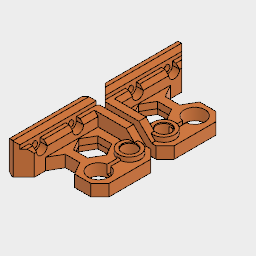
z_top_fix_v2.1 (Autodesk Fusion 360 design; units mm, degrees)
Autodesk Fusion 360 part; units mm, degrees
note: some values were not read from the file. Chosen so that the rebuilt part matches the saved one: which sketch regions a step uses; a direction; which face or edge a step refers to.
sketch "base_top_holes" plane through (0, 0, 0) normal (0, 0, 1) x (1, 0, 0)
  line L0 (0, 0) -> (38, 0)
  line L1 (38, 0) -> (38, 33)
  line L2 (8, 45) -> (0, 45)
  line L3 (0, 45) -> (0, 0)
  line L4 (8, 45) -> (8, 0)
  line L5 (8, 4) -> (30.5, 4)
  circle A0 centre (29.3, 8) radius 4
  circle A1 centre (16, 15) radius 7.7 construction
  circle A2 centre (16, 33) radius 8 construction
  circle A3 centre (29.3, 25) radius 5.75
  line L6 (16, 15) -> (16, 33) construction
  line L7 (29.3, 8) -> (29.3, 25) construction
  line L8 (20, 39.9282) -> (12, 39.9282)
  line L9 (12, 39.9282) -> (8, 33)
  line L10 (8, 33) -> (12, 26.0718)
  line L11 (12, 26.0718) -> (20, 26.0718)
  line L12 (20, 26.0718) -> (24, 33)
  line L13 (24, 33) -> (20, 39.9282)
  line L14 (23.7, 15) -> (19.85, 21.6684)
  line L15 (19.85, 21.6684) -> (12.15, 21.6684)
  line L16 (12.15, 21.6684) -> (8.3, 15)
  line L17 (8.3, 15) -> (12.15, 8.3316)
  line L18 (12.15, 8.3316) -> (19.85, 8.3316)
  line L19 (19.85, 8.3316) -> (23.7, 15)
  line L20 (28.3, 23) -> (30.3, 23)
  line L21 (30.3, 23) -> (30.3, 8)
  line L22 (30.3, 8) -> (28.3, 8)
  line L23 (28.3, 8) -> (28.3, 23)
  line L24 (30.5, 4) -> (30.5, 0)
  circle A4 centre (29.3, 8) radius 2.5
  line L25 (38, 33) -> (8, 33)
  line L26 (4, 0) -> (4, 45)
  point P0 (16, 33)
  point P1 (16, 15)
  dimension "d1" = 38
  dimension "d2" = 45
  dimension "d3" = 8
  dimension "d5" = 8
  dimension "d6" = 29.3
  dimension "d7" = 8
  dimension "d8" = 16
  dimension "d9" = 15
  dimension "d10" = 33
  dimension "d11" = 25
  dimension "d12" = 16
  dimension "d13" = 15.4
  dimension "d14" = 11.5
  dimension "d15" = 15
  dimension "d16" = 2
  dimension "d17" = 4
  dimension "d18" = 7.5
  dimension "d41" = 1.5
  measures "d1" distance of L0.start L0.end
  measures "d2" distance of L0.start L2.end
  measures "d3" distance of L2.end L2.start
  measures "d5" diameter of A0
  measures "d6" distance of L3 A0.centre
  measures "d7" distance of L0.start A0.centre
  measures "d8" distance of L0.start P1
  measures "d9" distance of L0.start P1
  measures "d10" distance of L0.start A2.centre
  measures "d11" distance of L0.start A3.centre
  measures "d12" diameter of A2
  measures "d13" diameter of A1
  measures "d14" diameter of A3
  measures "d15" distance of L20.end L21.end
  measures "d16" distance of L21.end L22.end
  measures "d17" distance of L5.end L24.end
  measures "d18" distance of L1 L24
  measures "d41" distance of A0 A4
extrude "Extrude1" add sketch "base_top_holes" against normal blind 6.5 contours L0 L2 L3 L26 | L0 L2 L4 L26 | L0 L4 L5 L24 | L0 L1 L4 L5 L10 L11 L12 L24 L25 makes body 1
extrude "Extrude2" add sketch "base_top_holes" along normal blind 11 contours L0 L2 L3 L26 bodies 1
extrude "Extrude3" add sketch "base_top_holes" along normal blind 7 contours L0 L2 L4 L26 | L0 L4 L5 L24 bodies 1
extrude "Extrude7" add sketch "base_top_holes" along normal blind 1.5 from surface at -6.5 contours A0 L21 L23 A4 | A0 A3 L21 L23 | A0 L21 L23 A4 bodies 1
sketch "frame_holes" plane through (0, 0, 0) normal (-1, 0, 0) x (0, -1, 0)
  line L0 (-45, 11) -> (-45, -6.5)
  line L1 (-45, -6.5) -> (0, -6.5)
  line L2 (0, -6.5) -> (0, 11)
  line L3 (0, 11) -> (-45, 11)
  line L4 (0, -6.5) -> (-45, -6.5)
  line L5 (0, -6.5) -> (0, 11)
  circle A0 centre (-15, 5) radius 3
  circle A1 centre (-35, 5) radius 3
  circle A2 centre (-35, 5) radius 1.65
  circle A3 centre (-15, 5) radius 1.65
  line L6 (-35, 5) -> (-15, 5) construction
  line L7 (0, 7) -> (-45, 7)
  line L8 (0, 7) -> (-45, 7)
  line L9 (-45, 7) -> (-45, 11)
  line L10 (-45, 11) -> (0, 11)
  line L11 (0, 11) -> (0, 7)
  line L12 (-38, 7) -> (-38, 5)
  line L13 (-32, 5) -> (-32, 7)
  line L14 (-18, 5) -> (-18, 7)
  line L15 (-12, 5) -> (-12, 7)
  line L16 (-35.825, 6.4289) -> (-35.4039, 6.85)
  line L17 (-35.4039, 6.85) -> (-34.5961, 6.85)
  line L18 (-34.5961, 6.85) -> (-34.175, 6.4289)
  line L19 (-15.825, 6.4289) -> (-15.4039, 6.85)
  line L20 (-15.4039, 6.85) -> (-14.5961, 6.85)
  line L21 (-14.5961, 6.85) -> (-14.175, 6.4289)
  line L22 (-35, 6.85) -> (-35, 5) construction
  line L23 (-15, 6.85) -> (-15, 5) construction
  dimension "d26" = 3.3
  dimension "d27" = 3.3
  dimension "d28" = 15
  dimension "d29" = 20
  dimension "d30" = 11.5
  dimension "d31" = 6
  dimension "d32" = 6
  dimension "d123" = 0.2
  dimension "d124" = 45
  dimension "d125" = 1.65
  dimension "d126" = 0.2
  dimension "d128" = 1.65
  measures "d26" diameter of A2
  measures "d27" diameter of A3
  measures "d28" distance of L1.end A0.centre
  measures "d29" distance of A0.centre A1.centre
  measures "d30" distance of L1.end A0.centre
  measures "d31" diameter of A1
  measures "d32" diameter of A0
  measures "d123" distance of A2 L17
  measures "d124" angle of L16 L17
  measures "d125" distance of L16.start L18.end
  measures "d126" distance of A3 L20
  measures "d128" distance of L19.start L21.end
extrude "Extrude5" cut sketch "frame_holes" against normal up to surface (8 mm away) contours A1 L7 L8 L12 | A1 L7 L8 | A1 L7 L8 | A0 L7 L8 L15 | A1 L7 L8 L13 | A0 L7 L8 | A0 L7 L8 | A0 L7 L8 L14 | A2 | A2 L16 L17 L18 | A3 | A3 L19 L20 L21 bodies 1
extrude "Extrude6" add sketch "frame_holes" against normal blind 4 contours A1 L7 L8 L12 | A1 L7 L8 | A1 L7 L8 | A0 L7 L8 L15 | A1 L7 L8 L13 | A0 L7 L8 | A0 L7 L8 | A0 L7 L8 L14 bodies 1
chamfer "Chamfer1" distance 2 angle 45 4 edges at (8, 8, 7) (8, 25, 7) (8, 41.5, 7) (4, 22.5, 11) on bodies 1
chamfer "Chamfer2" distance 7 angle 45 1 edges at (30.5, 2, 7) on bodies 1
chamfer "Chamfer3" distance 5 angle 45 2 edges at (38, 33, -3.25) (38, 0, -3.25) on bodies 1
chamfer "Chamfer4" distance 5.8 angle 45 1 edges at (8, 45, -0.75) on bodies 1
sketch "chamfer_line" plane through (0, 0, 0) normal (-1, 0, 0) x (0, -1, 0)
  line L0 (-45, 11) -> (-45, -6.5)
  line L1 (-45, -6.5) -> (0, -6.5)
  line L2 (0, -6.5) -> (0, 11)
  line L3 (0, 11) -> (-45, 11)
  line L4 (0, -6.5) -> (0, 11)
  line L5 (0, -6.5) -> (-45, -6.5)
  line L6 (-11.5, -6.5) -> (0, 5)
  arc A0 (-35.825, 6.4289) -> (-34.175, 6.4289) centre (-35, 5) ccw
  line L7 (-35.825, 6.4289) -> (-35.4039, 6.85)
  line L8 (-35.4039, 6.85) -> (-34.5961, 6.85)
  line L9 (-34.5961, 6.85) -> (-34.175, 6.4289)
  arc A1 (-15.825, 6.4289) -> (-14.175, 6.4289) centre (-15, 5) ccw
  line L10 (-15.825, 6.4289) -> (-15.4039, 6.85)
  line L11 (-15.4039, 6.85) -> (-14.5961, 6.85)
  line L12 (-14.5961, 6.85) -> (-14.175, 6.4289)
  dimension "d58" = 11.5
  dimension "d59" = 11.5
  measures "d58" distance of L1.end L6.start
  measures "d59" distance of L1.end L6.end
ref_plane "WorkPlane1" through (0, 5.75, -0.75) normal (-0.707107, 0.5, 0.5) x (0, -0.707107, 0.707107)
sketch "chamfer" plane through (0, 5.75, -0.75) normal (-0.707107, 0.5, 0.5) x (0, -0.707107, 0.707107)
  line L0 (0, -5.75) -> (12.3744, 3)
  line L1 (0, -5.75) -> (-31.8198, 16.75)
  line L2 (-8.1317, 0) -> (8.1317, 0)
  point P0 (8.1317, 0)
extrude "Extrude8" cut sketch "chamfer" against normal blind 30 bodies 1
sketch "rod_reinforcement" plane through (0, 0, 0) normal (0, 0, 1) x (-1, 0, 0)
  line L0 (-33, 0) -> (-38, -5)
  line L1 (-38, -5) -> (-38, -28)
  line L2 (-38, -28) -> (-33, -33)
  line L3 (-33, -33) -> (-24, -33)
  line L4 (-24, -33) -> (-20, -26.0718)
  line L5 (-20, -26.0718) -> (-12, -26.0718)
  line L6 (-12, -26.0718) -> (-8, -33)
  line L7 (-8, -33) -> (-8, -4)
  line L8 (-8.3, -15) -> (-12.15, -21.6684)
  line L9 (-12.15, -21.6684) -> (-19.85, -21.6684)
  line L10 (-19.85, -21.6684) -> (-23.7, -15)
  line L11 (-23.7, -15) -> (-19.85, -8.3316)
  line L12 (-19.85, -8.3316) -> (-12.15, -8.3316)
  line L13 (-12.15, -8.3316) -> (-8.3, -15)
  line L14 (-8, -4) -> (-29.3, -4)
  arc A0 (-28.3, -11.873) -> (-29.3, -4) centre (-29.3, -8) ccw
  line L15 (-28.3, -11.873) -> (-28.3, -19.3376)
  arc A1 (-30.3, -19.3376) -> (-28.3, -19.3376) centre (-29.3, -25) ccw
  line L16 (-30.3, -19.3376) -> (-30.3, -11.873)
  arc A2 (-29.3, -4) -> (-30.3, -11.873) centre (-29.3, -8) ccw
  line L17 (-30.5, -4) -> (-30.5, 0)
  line L18 (-30.5, 0) -> (-33, 0)
  arc A3 (-30.3, -19.3376) -> (-28.3, -19.3376) centre (-29.3, -25) ccw
  line L19 (-38, -5) -> (-38, -28)
  circle A4 centre (-29.3, -8) radius 6
  line L20 (-30.3, -19.3376) -> (-30.3, -11.873)
  line L21 (-28.3, -11.873) -> (-28.3, -19.3376)
  arc A5 (-28.3, -11.873) -> (-29.3, -4) centre (-29.3, -8) ccw
  arc A6 (-29.3, -4) -> (-30.3, -11.873) centre (-29.3, -8) ccw
  circle A7 centre (-29.3, -8) radius 2.5
  arc A8 (-30.3, -11.873) -> (-28.3, -11.873) centre (-29.3, -8) ccw
  line L22 (-29.3, -4) -> (-30.5, -4)
  dimension "d76" = 12
  measures "d76" diameter of A4
extrude "Extrude11" add sketch "rod_reinforcement" along normal blind 2.5 contours L14 L17 A4 L22 | L16 A2 L17 A4 L20 A6 L22 | L14 A0 L15 A4 L21 A5 bodies 1
extrude "Extrude12" add sketch "rod_reinforcement" against normal blind 1.6 from surface at 2.5 contours L14 L17 A4 L22 | L15 L16 A4 L20 L21 A8 bodies 1
chamfer "Chamfer11" distance 0.5 distance2 0.15 1 edges at (29.7682, 4.0275, 2.5) measured on face at (30.6677, 11.7589, 1.1333) on bodies 1
chamfer "Chamfer6" distance 5 angle 45 1 edges at (0, 0, 8) on bodies 1
chamfer "Chamfer9" distance 1.5 angle 45 1 edges at (0, 28.25, -6.5) on bodies 1
chamfer "Chamfer10" distance 0.26 distance2 3 6 edges at (10.225, 18.3342, -6.5) (10.225, 11.6658, -6.5) (16, 8.3316, -6.5) (21.775, 11.6658, -6.5) (21.775, 18.3342, -6.5) (16, 21.6684, -6.5) measured on face at (3.6667, 29.1262, -6.5) measured on face at (3.6667, 29.1262, -6.5) measured on face at (3.6667, 29.1262, -6.5) measured on face at (3.6667, 29.1262, -6.5) measured on face at (3.6667, 29.1262, -6.5) measured on face at (3.6667, 29.1262, -6.5) on bodies 1
sketch "selective_infill" plane through (0, 0, -6.5) normal (0, 0, -1) x (1, 0, 0)
  circle A0 centre (29.3, -8) radius 2.5
  circle A1 centre (29.3, -25) radius 5.75
  line L0 (1.5, -9.3787) -> (1.5, -45)
  line L1 (1.5, -45) -> (2.2, -45)
  line L2 (2.2, -45) -> (8, -39.2)
  line L3 (8, -39.2) -> (8, -33)
  line L4 (8, -33) -> (12, -26.0718)
  line L5 (12, -26.0718) -> (20, -26.0718)
  line L6 (20, -26.0718) -> (24, -33)
  line L7 (24, -33) -> (33, -33)
  line L8 (33, -33) -> (38, -28)
  line L9 (38, -28) -> (38, -5)
  line L10 (38, -5) -> (33, 0)
  line L11 (33, 0) -> (8.1317, 0)
  line L12 (8.1317, 0) -> (1.5, -9.3787)
  line L13 (20.0001, -8.0716) -> (24.0002, -15)
  line L14 (24.0002, -15) -> (20.0001, -21.9284)
  line L15 (20.0001, -21.9284) -> (11.9999, -21.9284)
  line L16 (11.9999, -21.9284) -> (7.9998, -15)
  line L17 (7.9998, -15) -> (11.9999, -8.0716)
  line L18 (11.9999, -8.0716) -> (20.0001, -8.0716)
  line L19 (12.15, -8.3316) -> (19.85, -8.3316)
  line L20 (38, -28) -> (38, -5)
  line L21 (33, 0) -> (8.1317, 0)
  line L22 (12, -26.0718) -> (20, -26.0718)
  line L23 (19.85, -21.6684) -> (12.15, -21.6684)
  circle A2 centre (29.3, -25) radius 5.75
  line L24 (8, -33) -> (8, -4)
  line L25 (8, -4) -> (24.8279, -4)
  line L26 (6.3, -23.8196) -> (21.05, -23.8196)
  line L27 (21.05, -23.8196) -> (21.05, -23.9206)
  line L28 (21.05, -23.9206) -> (6.3, -23.9206)
  line L29 (6.3, -23.9206) -> (6.3, -23.8196)
  line L30 (7.55, -1.9495) -> (28, -1.9495)
  line L31 (28, -1.9495) -> (28, -2.0505)
  line L32 (28, -2.0505) -> (7.55, -2.0505)
  line L33 (7.55, -2.0505) -> (7.55, -1.9495)
  line L34 (35.399, -7.5) -> (35.5, -7.5)
  line L35 (35.5, -7.5) -> (35.5, -19.4444)
  line L36 (35.5, -19.4444) -> (35.399, -19.4444)
  line L37 (35.399, -19.4444) -> (35.399, -7.5)
  line L38 (16, -26.0718) -> (16, -21.6684) construction
  line L39 (21.05, -23.8701) -> (16, -23.8701) construction
  circle A3 centre (29.3, -8) radius 2.5
  line L40 (38, -5) -> (38, -28)
  line L41 (16.4139, -4) -> (16.4139, 0) construction
  line L42 (28, -2) -> (16.4139, -2) construction
  line L43 (30.5, -2.1212) -> (30.5, 0)
  dimension "d97" = 2.5
  dimension "d98" = 0.101
  dimension "d99" = 1.7
  dimension "d102" = 2.5
  dimension "d104" = 2.5
  dimension "d105" = 0.101
  dimension "d107" = 0.101
  dimension "d109" = 0.45
  dimension "d120" = 2.5
  dimension "d129" = 2.5
  measures "d97" distance of A2 L27
  measures "d98" distance of L26.end L27.end
  measures "d99" distance of L24 L28.end
  measures "d102" distance of A1 L36.end
  measures "d104" distance of L9.end L34
  measures "d105" distance of L34.start L34.end
  measures "d107" distance of L30.end L31.end
  measures "d109" distance of L24.end L33
  measures "d120" distance of L31 L43.end
  measures "d129" distance of L9 L35
extrude "Extrude14" cut sketch "selective_infill" against normal up to surface (2.5 mm away) from surface at -2 contours L24 L26 L28 L29 | L24 L26 L27 L28 | L30 L31 L32 L33 | L34 L35 L36 L37 bodies 1
extrude "Extrude15" cut sketch "selective_infill" against normal up to surface (5.7 mm away) from surface at -1 contours L30 L31 L32 L33 bodies 1
mirror "Mirror2" about plane through (0, 0, 0) normal (0, 1, 0) of bodies 1 makes body 2
move_body "Move2" bodies 2 to x (1, 0, 0) y (0, 1, 0) z (0, 0, 1) at (0, -3, 0)
equation "d5 = rod_dia"
equation "d26 = m3_hole"
equation "d27 = m3_hole"
equation "d31 = m3_head"
equation "d32 = m3_head"
equation "rod_dia = 8.00 mm"
equation "layer_height = 0.2 mm"
equation "extrusion_width = 0.45 mm"
equation "num_perimeters = 3"
equation "num_tops_bottoms = 5"
equation "perimeters_thickness = num_perimeters * extrusion_width - 0.1 mm"
equation "top_bottom_thickness = num_tops_bottoms * layer_height"
equation "d97 = perimeters_thickness * 2"
equation "d99 = perimeters_thickness + extrusion_width"
equation "d102 = perimeters_thickness * 2"
equation "d104 = perimeters_thickness * 2"
equation "d109 = extrusion_width"
equation "d114 = -top_bottom_thickness * 2"
equation "d115 = -top_bottom_thickness * 2"
equation "d117 = -top_bottom_thickness"
equation "d118 = layer_height"
equation "d120 = perimeters_thickness * 2"
equation "m3_hole = 3.3 mm"
equation "m3_head = 6 mm"
equation "d123 = layer_height"
equation "d125 = m3_hole / 2"
equation "d126 = layer_height"
equation "d128 = m3_hole / 2"
equation "d129 = perimeters_thickness * 2"
named bodies: "z_top_fix_right", "z_top_fix_left"
